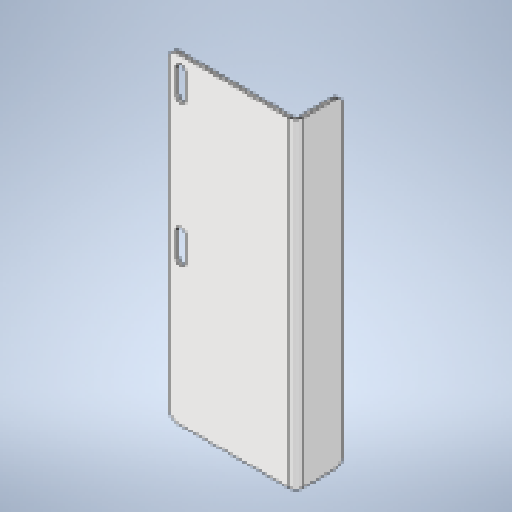
# Autodesk Inventor part: GNH 017  Pulse compensator
Saved by Autodesk Inventor 2025.1 (Build 291241020, 241B)
## iProperties
Created: 2023-03-28
Part Number: GNH 017  Pulse compensator
Material: Stainless Steel
Description: bend
Document SubType Name: Sheet Metal
Designer: user
Stock Number: bend
Mass: 337.2 g
Surface Area: 435.517 cm^2
Volume: 42.1501 cm^3
Density: 8 g/cm^3
Flat Pattern Width: 20 cm
Flat Pattern Length: 10.6524 cm
Flat Pattern Area: 213.048 cm^2
Sheet Metal Rule: Default_mm
Sheet Metal Width: 200.000 mm
Sheet Metal Length: 106.524 mm
Sheet Metal Area: 21304.779 mm^2
Appearance: Default
Author: user
Autodesk Inventor part; units mm, degrees
ref_plane "YZ Plane" through (0, 0, 0) normal (1, 0, 0) x (0, 1, 0)
ref_plane "XZ Plane" through (0, 0, 0) normal (0, 1, 0) x (-1, 0, 0)
ref_plane "XY Plane" through (0, 0, 0) normal (0, 0, 1) x (1, 0, 0)
sketch "Sketch1" plane through (0, 0, 0) normal (0, 0, 1) x (1, 0, 0)
  line L0 (40, -100) -> (-40, -100)
  line L1 (-40, -100) -> (-40, 100)
  line L2 (-40, 100) -> (40, 100)
  line L3 (40, 100) -> (40, -100)
  line L4 (40, 100) -> (-40, -100) construction
  point P0 (0, 0)
  point P1 (0, 0)
  dimension "d1" = 200
  dimension "d2" = 80
  constraints: 10 end point, 2 parallel, 1 coincident, 1 horizontal, 1 midpoint, 1 perpendicular
  measures "d1" distance of L2.end L0.start
  measures "d2" distance of L1.end L2.end
extrude "Plate1" add sketch "Sketch1" along normal blind 2
sketch "Sketch5" plane through (0, 0, 0) normal (0, 0, 1) x (1, 0, 0)
  circle A0 centre (-32, 92) radius 3
  circle A1 centre (-32, 4) radius 3
  line L0 (-40, -100) -> (-40, 100) projected
  line L1 (40, -100) -> (-40, -100) projected
  line L2 (40, 100) -> (40, -100) projected
  line L3 (-40, 100) -> (40, 100) projected
  line L4 (-32, 92) -> (-32, 77) construction
  line L5 (-35, 92) -> (-35, 77)
  line L6 (-29, 77) -> (-29, 92)
  arc A2 (-29, 92) -> (-35, 92) centre (-32, 92) ccw
  arc A3 (-35, 77) -> (-29, 77) centre (-32, 77) ccw
  line L7 (-32, 4) -> (-32, -11) construction
  line L8 (-35, 4) -> (-35, -11)
  line L9 (-29, -11) -> (-29, 4)
  arc A4 (-29, 4) -> (-35, 4) centre (-32, 4) ccw
  arc A5 (-35, -11) -> (-29, -11) centre (-32, -11) ccw
  point P0 (0, 0)
  point P1 (-32, 84.5)
  point P2 (-32, -3.5)
  point P3 (-29, 4)
  dimension "d33" = 88
  dimension "d34" = 6
  dimension "d35" = 8
  dimension "d36" = 8
  dimension "d50" = 15
  constraints: 16 end point, 8 point on circle, 8 tangent, 6 centre point, 3 equal radius, 2 midpoint, 2 parallel, 2 vertical, 1 collinear, 1 vertical alignment
  measures "d33" distance of L7.start L4.start
  measures "d34" diameter of A1
  measures "d35" distance from line of L3 L4.start
  measures "d36" distance from line of L0 L4.start
  measures "d50" distance of L7.start L7.end
extrude "Cut1" cut sketch "Sketch5" along normal blind 2 contours A0 | L6 A3 L5 A0 | A1 | L9 A5 L8 A1
sketch "Sketch6" plane through (38, 100, 2) normal (1, 0, 0) x (0, 1, 0)
  line L0 (-200, 0) -> (0, 0)
  line L1 (0, 0) -> (0, 30)
  line L2 (0, 30) -> (-200, 30)
  line L3 (-200, 30) -> (-200, 0)
  constraints: 6 end point, 1 horizontal, 1 perpendicular, 1 vertical
edge flange "Flange2" height 30 angle 90 thickness 2 bend radius 2 thickness toward (1, 0, 0) relief tear relief width 2 relief depth 1 edges at (40, 0, 2) wall of the first edge with corners at (38, -100, 2) (38, 100, 2) (38, 100, -28) (38, -100, -28)
bend "Bend2"
corner "Corner2"
fillet "Corner Round1" radius 6 4 edges at (-40, 100, 1) (39, -100, -28) (39, 100, -28) (-40, -100, 1)
equation "\"d36\" = d35"
equation "\"d37\" = Thickness"
equation "\"d0\" = Thickness"
equation "\"d39\" = BendReliefWidth"
equation "\"d40\" = BendReliefDepth"
equation "\"d41\" = MinimumRemnant"
equation "\"d42\" = TransitionRadius"
equation "\"d45\" = BendRadius"
equation "\"d46\" = CornerReliefSize"
equation "\"d47\" = GapSize"
equation "\"d48\" = JacobiRadiusSize"
equation "\"BendRadius\" = Thickness"
equation "\"BendReliefWidth\" = Thickness"
equation "\"BendReliefDepth\" = 0.5 * Thickness"
equation "\"CornerReliefSize\" = 4 * Thickness"
equation "\"MinimumRemnant\" = 2 * Thickness"
equation "\"TransitionRadius\" = BendRadius"
equation "\"JacobiRadiusSize\" = BendRadius"
equation "\"GapSize\" = Thickness"
equation "\"Thickness\" = 2"
body "Solid1"
